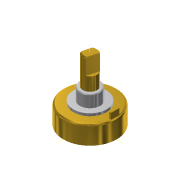
# Autodesk Inventor part: empty
Saved by Autodesk Inventor 2014 (Build 180170000, 170)
## iProperties
Created: 2015-04-13
Part Number: empty
Material: Generic
Document SubType Name: Modeling
Designer: Martin
Density: 1 g/cm^3
Appearance: Default
Author: Martin
Autodesk Inventor part; units mm, degrees
ref_plane "YZ Plane" through (0, 0, 0) normal (1, 0, 0) x (0, 1, 0)
ref_plane "XZ Plane" through (0, 0, 0) normal (0, 1, 0) x (-1, 0, 0)
ref_plane "XY Plane" through (0, 0, 0) normal (0, 0, 1) x (1, 0, 0)
sketch "Sketch1" plane through (0, 0, 0) normal (1, 0, 0) x (0, 1, 0)
  line L0 (0, -3.04) -> (0, 18.24) projected
  line L1 (-1.3, 0) -> (7.8, 0) projected
  line L2 (6.5, 0) -> (6.5, 4.5)
  line L3 (6.5, 4.5) -> (4.03, 4.5)
  line L4 (4.03, 4.5) -> (4.03, 5.1)
  line L5 (4.03, 5.1) -> (2.5, 5.1)
  line L6 (2.5, 5.1) -> (2.5, 8.05)
  line L7 (2.5, 8.05) -> (1.75, 8.05)
  line L8 (1.75, 8.05) -> (1.75, 15.2)
  line L9 (1.75, 15.2) -> (0, 15.2)
  line L10 (6.5, 0) -> (0, 0)
  line L11 (0, 0) -> (0, 15.2)
  dimension "d0" = 4.5
  dimension "d1" = 5.1
  dimension "d2" = 8.05
  dimension "d3" = 10.1
  dimension "d4" = 13
  dimension "d5" = 8.06
  dimension "d6" = 5
  dimension "d7" = 3.5
  constraints: 20 end point, 6 parallel, 4 perpendicular, 2 point on line
  measures "d0" distance of L2.start L2.end
  measures "d1" distance between parallel lines of L1 L5
  measures "d2" distance between parallel lines of L1 L7
  measures "d3" distance between parallel lines of L5 L9
  measures "d4" diameter of L2 L0
  measures "d5" diameter of L4 L0
  measures "d6" diameter of L6 L0
  measures "d7" diameter of L8 L0
revolve "Revolution1" add sketch "Sketch1" angle 360 about axis through (0, 0, -10) along (0, 0, 1)
fillet "Fillet1" radius 0.5 1 edges at (0, -6.5, 4.5)
fillet "Fillet2" radius 0.3 1 edges at (0, -2.5, 8.05)
sketch "Sketch2" plane through (0, 0, 0) normal (1, 0, 0) x (0, 1, 0)
  line L0 (-6.5, 0) -> (6.5, 0) projected
  line L1 (3.5, 0) -> (3.8, 0)
  line L2 (3.8, 0) -> (3.8, -0.6)
  line L3 (3.8, -0.6) -> (-2.2, -0.8095)
  line L4 (-2.2, -0.8095) -> (-2.2, -0.5093)
  line L5 (-2.2, -0.5093) -> (3.5, -0.3103)
  line L6 (3.5, -0.3103) -> (3.5, 0)
  arc A0 (3.1899, -0.3211) -> (3.5, 0) centre (3.1787, 0) ccw
  arc A1 (3.4899, -0.6108) -> (3.8, -0.2897) centre (3.4787, -0.2897) ccw
  point P0 (0, 0)
  dimension "d11" = 0.6
  dimension "d12" = 92
  dimension "d13" = 0.3
  dimension "d14" = 0.3
  dimension "d15" = 2.7
  dimension "d16" = 6
  constraints: 12 end point, 5 point on line, 4 point on circle, 4 tangent, 3 parallel, 2 centre point, 1 equal radius, 1 perpendicular
  measures "d11" distance of L1.end L2.end
  measures "d12" angle of L6 L5
  measures "d13" distance between parallel lines of L2 L6
  measures "d14" distance between parallel lines of L3 L5
  measures "d15" horizontal distance of A1.end L0.end
  measures "d16" horizontal distance of L2.end L3.end
extrude "Extrusion1" add sketch "Sketch2" along normal mid plane 0.7 contours L0 L2 A1 L3 L4 L5 L6
pattern_linear "Rectangular Pattern1" count 3 spacing 2.54 along (1, 0, 0) of "Extrusion1" first direction both ways yes
sketch "Sketch3" plane through (0, 0, 15.2) normal (0, 0, 1) x (1, 0, 0)
  circle A0 centre (0, 0) radius 1.75 projected
  line L0 (0, -9.1) -> (0, 9.1) projected
  line L1 (-0.4529, -1.6904) -> (0.4529, 1.6904) construction
  line L2 (-1.3376, -1.1284) -> (-0.5942, 1.646)
  line L3 (0.5942, -1.646) -> (1.3376, 1.1284)
  dimension "d22" = 15
  dimension "d23" = 2
  constraints: 6 end point, 6 point on circle, 1 coincident, 1 midpoint, 1 parallel, 1 other
  measures "d22" angle of L0 L1
  measures "d23" distance between parallel lines of L3 L2
extrude "Extrusion2" cut sketch "Sketch3" against normal blind 3.9 contours A0 L3 | L2 A0
chamfer "Chamfer1" distance 0.3 angle 45 3 edges at (-0.3016, 1.7238, 15.2) (0.7375, 1.587, 15.2) (-0.4529, -1.6904, 15.2)
sketch "Sketch4" plane through (0, 0, 0) normal (0, 1, 0) x (-1, 0, 0)
  line L0 (-6.5, 4) -> (-6.5, 0) projected
  arc A0 (-6, 4.5) -> (-6.5, 4) centre (-6, 4) ccw projected
  line L1 (-4.03, 4.5) -> (4.03, 4.5) projected
  line L2 (-6, 4.5) -> (6, 4.5) projected
  line L3 (-6.15, 4.477) -> (-6.15, 5.95)
  line L4 (-6.15, 5.95) -> (-5.75, 5.95)
  line L5 (-5.75, 5.95) -> (-5.75, 4.5)
  arc A1 (-6, 4.5) -> (-6.15, 4.477) centre (-6, 4) ccw
  line L6 (-6, 4.5) -> (-5.75, 4.5)
  point P0 (0, 0)
  dimension "d29" = 0.4
  dimension "d31" = 0.35
  dimension "d32" = 1.45
  constraints: 8 end point, 5 point on circle, 3 tangent, 2 perpendicular, 1 centre point, 1 collinear, 1 concentric, 1 parallel, 1 point on line
  measures "d29" distance of L3.end L4.end
  measures "d31" distance between parallel lines of L3 L0
  measures "d32" distance of L4.end L5.end
extrude "Extrusion3" add sketch "Sketch4" along normal mid plane 2
body "Solid1"
